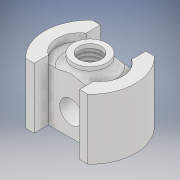
# Autodesk Inventor part: Crosshead
Saved by Autodesk Inventor 2017 (Build 210142000, 142)
## iProperties
Created: 2018-11-11
Part Number: Crosshead
Material: Copper, Wrought
Document SubType Name: Modeling
Designer: Arman Grewal
Density: 8.94 g/cm^3
Appearance: Snow
Author: Arman Grewal
Autodesk Inventor part; units mm, degrees
ref_plane "XZ Plane" through (0, 0, 0) normal (0, 1, 0) x (-1, 0, 0)
ref_plane "XY Plane" through (0, 0, 0) normal (0, 0, 1) x (1, 0, 0)
sketch "Sketch1" plane through (0, 0, 0) normal (0, 1, 0) x (-1, 0, 0)
  circle A0 centre (0, 0) radius 12 construction
  line L0 (-5, -16.2951) -> (5, -16.2951) construction
  arc A1 (-8.75, -8.212) -> (8.75, -8.212) centre (0, 0) ccw construction
  arc A2 (-8.75, -8.212) -> (8.75, -8.212) centre (0, 0) ccw
  line L1 (14.6502, 6) -> (14.6502, -6) construction
  line L2 (8.75, -8.212) -> (8.75, -6)
  line L3 (8.75, -6) -> (5, -6)
  line L4 (-8.75, -8.212) -> (-8.75, -6)
  line L5 (-8.75, -6) -> (-5, -6)
  arc A3 (-5, -6) -> (5, -6) centre (0, -2.6834) ccw
  line L6 (14.6502, 0) -> (-10.8345, 0) construction
  line L7 (8.75, -8.212) -> (8.75, 12.1901) construction
  line L8 (-8.75, -8.212) -> (-8.75, 14.7434) construction
  arc A4 (8.75, 8.212) -> (-8.75, 8.212) centre (0, 0) ccw construction
  line L9 (8.75, 8.212) -> (8.75, 6) construction
  arc A5 (8.75, 8.212) -> (-8.75, 8.212) centre (0, 0) ccw
  line L10 (8.75, 8.212) -> (8.75, 6)
  line L11 (-8.75, 8.212) -> (-8.75, 7.106)
  line L12 (-8.75, 7.106) -> (-8.75, 6)
  line L13 (-8.75, 6) -> (-5, 6)
  line L14 (8.75, 6) -> (5, 6)
  arc A6 (5, 6) -> (-5, 6) centre (0, 2.6834) ccw
  line L15 (-5, 6) -> (-5, -6)
  line L16 (5, 6) -> (5, -6)
  circle A7 centre (0, 0) radius 4.75 construction
  circle A8 centre (0, 0) radius 3 construction
  point P0 (0, -16.2951)
  dimension "d0" = 24
  dimension "d1" = 10
  dimension "d2" = 12
  dimension "d3" = 6
  dimension "d4" = 6
  dimension "d5" = 9.5
  dimension "d6" = 6
  constraints: 34 end point, 16 point on circle, 9 centre point, 5 point on line, 5 vertical, 4 concentric, 4 horizontal, 3 coincident, 2 midpoint, 2 perpendicular, 1 collinear, 1 horizontal alignment, 1 parallel, 1 vertical alignment
  measures "d0" diameter of A0
  measures "d1" distance of L0.start L0.end
  measures "d2" distance of L1.start L1.end
  measures "d3" radius of A3
  measures "d4" radius of A6
  measures "d5" diameter of A7
  measures "d6" diameter of A8
extrude "Extrusion1" add sketch "Sketch1" along normal blind 16
sketch "Sketch2" plane through (0, 16, 0) normal (0, 1, 0) x (1, 0, 0)
  line L0 (-5, 6) -> (-5, -6) projected
  line L1 (-5, -6) -> (-5, 6)
  line L2 (5, -6) -> (5, 6) projected
  line L3 (5, -6) -> (5, 6)
  arc A0 (-5, -6) -> (5, -6) centre (0, -2.6834) ccw
  line L4 (5, 6) -> (8.75, 6) projected
  arc A1 (5, 6) -> (-5, 6) centre (0, 2.6834) ccw
  point P0 (0, 0)
  dimension "d9" = 6
  dimension "d10" = 6
  constraints: 4 end point, 4 point on circle, 2 centre point, 1 collinear, 1 vertical
  measures "d9" radius of A0
  measures "d10" radius of A1
extrude "Extrusion2" cut sketch "Sketch2" against normal blind 2
sketch "Sketch3" plane through (0, 14, 0) normal (0, 1, 0) x (1, 0, 0)
  circle A0 centre (0, 0) radius 4.5
  circle A1 centre (0, 0) radius 3
  dimension "d13" = 9
  dimension "d14" = 6
  constraints: 2 centre point, 2 coincident
  measures "d13" diameter of A0
  measures "d14" diameter of A1
extrude "Extrusion3" add sketch "Sketch3" along normal blind 3
fillet "Fillet1" radius 2 1 edges at (-4.5, 14, 0)
ref_plane "Work Plane1" through (14.75, 0, 0) normal (1, 0, 0) x (0, 1, 0)
sketch "Sketch4" plane through (14.75, 0, 0) normal (1, 0, 0) x (0, 1, 0)
  circle A0 centre (6, 0) radius 3
  point P0 (0, 0)
  dimension "d19" = 6
  dimension "d20" = 6
  constraints: 1 centre point, 1 horizontal alignment
  measures "d19" diameter of A0
  measures "d20" distance of A0.centre point (0, 0)
extrude "Extrusion4" cut sketch "Sketch4" against normal blind 888
sketch "Sketch5" plane through (0, 14, 0) normal (0, 1, 0) x (1, 0, 0)
  circle A0 centre (0, 0) radius 3
  dimension "d23" = 6
  constraints: 1 centre point, 1 coincident
  measures "d23" diameter of A0
extrude "Extrusion5" cut sketch "Sketch5" against normal up to surface round surface about axis through (14.75, 6, 0) along (-1, 0, 0) radius 3 far side no
thread "Thread2" size "M6" standard "Din Taper" length 10
body "Solid1"
